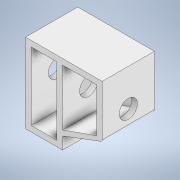
# Autodesk Inventor part: zmotorblock
Saved by Autodesk Inventor 2020 (Build 240168000, 168)
## iProperties
Created: 2020-11-21
Part Number: zmotorblock
Material: ABS Plastic
Document SubType Name: Modeling
Designer: AOB
Mass: 81.076 g
Surface Area: 328.673 cm^2
Volume: 76.4868 cm^3
Density: 1.06 g/cm^3
Appearance: Smooth - White
Author: AOB
Autodesk Inventor part; units mm, degrees
ref_plane "YZ Plane" through (0, 0, 0) normal (1, 0, 0) x (0, 1, 0)
ref_plane "XZ Plane" through (0, 0, 0) normal (0, 1, 0) x (-1, 0, 0)
sketch "Sketch1" plane through (0, 0, 0) normal (0, 0, 1) x (1, 0, 0)
  line L0 (-16.4376, 53.6188) -> (-16.4376, -6.3812)
  line L1 (16.1624, 3.9921) -> (16.1624, 53.6188)
  line L2 (16.0624, -11.3812) -> (-16.4376, -11.3812)
  line L3 (-16.4376, 58.6188) -> (48.5624, 58.6188)
  line L4 (-16.4376, 58.6188) -> (-16.4376, -11.3812)
  line L5 (-11.4376, 53.6188) -> (-11.4376, -6.3812)
  line L6 (11.1624, 53.6188) -> (11.1624, -6.3812)
  line L7 (43.5624, 53.6188) -> (46.1624, 53.6188)
  line L8 (11.1624, 53.6188) -> (-11.4376, 53.6188)
  line L9 (-11.4376, -6.3812) -> (11.1624, -6.3812)
  line L10 (18.7626, 0.4857) -> (43.5624, 9.7508)
  line L11 (16.1624, -1.8735) -> (16.1624, -11.3812)
  arc A0 (17.4625, 0) -> (16.1624, -1.8735) centre (18.1624, -1.8735) ccw
  line L12 (16.1624, -11.3812) -> (16.0624, -11.3812)
  line L13 (16.1624, 53.6188) -> (43.5624, 53.6188)
  line L14 (46.1624, 53.6188) -> (46.1624, 14.6188)
  line L15 (46.1624, 10.7222) -> (43.5624, 9.7508)
  line L16 (51.1624, 32.1705) -> (51.1624, 58.6188)
  line L17 (51.1624, 58.6188) -> (48.5624, 58.6188)
  line L18 (51.1624, 32.1705) -> (51.1624, 13.978)
  arc A1 (49.8624, 12.1045) -> (51.1624, 13.978) centre (49.1624, 13.978) ccw
  line L19 (46.1624, 14.6188) -> (16.1624, 3.9921)
  line L20 (17.4625, 0) -> (49.8624, 12.1045)
  point P0 (49.8624, 12.1045)
  point P1 (51.1624, 13.978)
  point P2 (16.1624, -1.8735)
  point P3 (17.4625, 0)
  point P4 (18.7626, 0.4857)
  point P5 (46.1624, 10.7222)
  constraints: 42 end point, 4 point on circle, 2 centre point
extrude "Extrusion5" add sketch "Sketch1" along normal blind 41
sketch "Sketch7" plane through (0, 0, 0) normal (0, 0, -1) x (-1, 0, 0)
  line L0 (16.4376, 58.6188) -> (16.4376, -11.3812) projected
  line L1 (16.4376, 58.6188) -> (16.4376, -11.3812)
  line L2 (-16.1624, -11.3812) -> (-16.1624, -1.8735) projected
  line L3 (16.4376, -11.3812) -> (-16.1624, -11.3812)
  line L4 (-16.1624, -11.3812) -> (-16.1624, 0.8571)
  line L5 (-51.1624, 58.6188) -> (16.4376, 58.6188) projected
  line L6 (16.4376, 58.6188) -> (-51.1624, 58.6188)
  arc A0 (-51.1624, 13.978) -> (-49.8624, 12.1045) centre (-49.1624, 13.978) ccw projected
  line L7 (-51.1624, 58.6188) -> (-51.1624, 13.978)
  line L8 (-17.4625, 0) -> (-49.8624, 12.1045) projected
  line L9 (-49.8624, 12.1045) -> (-17.4625, 0)
  arc A1 (-16.1624, -1.8735) -> (-17.4625, 0) centre (-18.1624, -1.8735) ccw
  arc A2 (-51.1624, 13.978) -> (-49.8624, 12.1045) centre (-49.1624, 13.978) ccw
  point P0 (0, 0)
  point P1 (-16.1624, -1.8735)
  constraints: 12 end point, 4 point on circle, 3 perpendicular, 2 centre point, 2 collinear, 1 coincident, 1 horizontal, 1 point on line, 1 tangent
extrude "Extrusion6" add sketch "Sketch7" along normal blind 5
ref_plane "Work Plane11" through (0, 0, 18) normal (0, 0, 1) x (1, 0, 0)
sketch "Sketch8" plane through (-11.4376, -6.3812, 41) normal (1, 0, 0) x (0, 0, -1)
  line L0 (46, 65) -> (0, 65) construction
  line L1 (46, 65) -> (0, 0) construction
  line L2 (46, -5) -> (46, 65) construction
  line L3 (0, 65) -> (0, -5) construction
  line L4 (46, 0) -> (0, 65) construction
  circle A0 centre (23, 32.5) radius 8
  circle A1 centre (23, 32.5) radius 9
  point P0 (41, 6.3812)
  dimension "d36" = 16
  dimension "d37" = 18
  constraints: 4 end point, 2 centre point, 1 coincident, 1 midpoint, 1 point on line
  measures "d36" diameter of A0
  measures "d37" diameter of A1
hole "Hole2" at (-11.4376, 26.1188, 18) direction (-1, 0, 0) diameter 16 end through all
hole "Hole3" at (-11.4376, 26.1188, 18) direction (1, 0, 0) diameter 16 end through all
body "Solid2"
